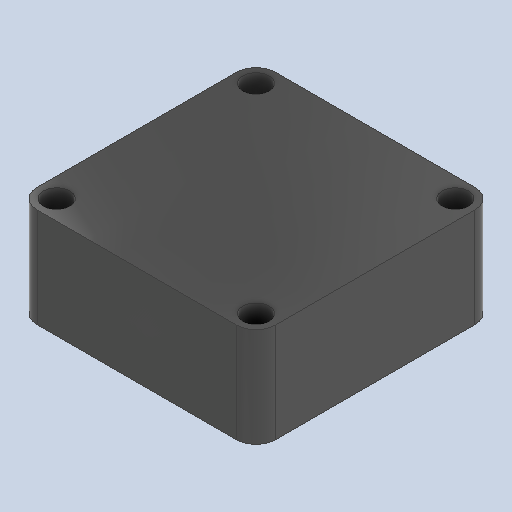
# Autodesk Inventor part: FC
Saved by Autodesk Inventor 2025.2 (Build 292293000, 293)
## iProperties
Created: 2025-03-28
Part Number: FC
Material: Generic
Document SubType Name: Modeling
Designer: mirewn
Density: 1 g/cm^3
Appearance: Default
Author: mirewn
Autodesk Inventor part; units mm, degrees
ref_plane "YZ Plane" through (0, 0, 0) normal (1, 0, 0) x (0, 1, 0)
ref_plane "XZ Plane" through (0, 0, 0) normal (0, 1, 0) x (-1, 0, 0)
ref_plane "XY Plane" through (0, 0, 0) normal (0, 0, 1) x (1, 0, 0)
sketch "Sketch1" plane through (0, 0, 0) normal (0, 1, 0) x (-1, 0, 0)
  line L0 (-15.05, 18) -> (15.05, 18)
  line L1 (18, 15.05) -> (18, -15.05)
  line L2 (15.05, -18) -> (-15.05, -18)
  line L3 (-18, -15.05) -> (-18, 15.05)
  line L4 (-18, 18) -> (18, -18) construction
  line L5 (18, 18) -> (-18, -18) construction
  circle A0 centre (15.05, 15.05) radius 2
  circle A1 centre (-15.05, 15.05) radius 2
  circle A2 centre (-15.05, -15.05) radius 2
  circle A3 centre (15.05, -15.05) radius 2
  arc A4 (18, 15.05) -> (15.05, 18) centre (15.05, 15.05) ccw
  arc A5 (15.05, -18) -> (18, -15.05) centre (15.05, -15.05) ccw
  arc A6 (-18, -15.05) -> (-15.05, -18) centre (-15.05, -15.05) ccw
  arc A7 (-15.05, 18) -> (-18, 15.05) centre (-15.05, 15.05) ccw
  point P0 (0, 0)
  dimension "d0" = 36
  dimension "d1" = 36
  dimension "d2" = 4
  dimension "d3" = 15.05
  dimension "d6" = 360
  dimension "d8" = 2.95
  constraints: 12 end point, 9 point on line, 8 centre point, 8 point on circle, 8 tangent, 3 equal radius, 2 midpoint, 2 parallel, 1 horizontal, 1 perpendicular, 9 other
  measures "d0" distance of L4.end L5.end
  measures "d1" distance of L5.start L4.end
  measures "d2" diameter of A0
  measures "d3" horizontal distance of point (0, 0) A0.centre
  measures "d8" radius of A4
extrude "Extrusion1" add sketch "Sketch1" along normal blind 15
body "Solid1"
